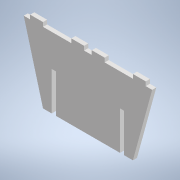
# Autodesk Inventor part: Base_Soporte
Saved by Autodesk Inventor 2022 (Build 260153000, 153)
## iProperties
Created: 2022-02-08
Part Number: Base_Soporte
Material: Generic
Document SubType Name: Modeling
Designer: katha
Density: 1 g/cm^3
Appearance: Default
Author: katha
Autodesk Inventor part; units mm, degrees
ref_plane "YZ Plane" through (0, 0, 0) normal (1, 0, 0) x (0, 1, 0)
ref_plane "XZ Plane" through (0, 0, 0) normal (0, 1, 0) x (-1, 0, 0)
ref_plane "XY Plane" through (0, 0, 0) normal (0, 0, 1) x (1, 0, 0)
sketch "Sketch1" plane through (0, 0, 0) normal (0, 0, 1) x (1, 0, 0)
  line L0 (49.5311, 184.3064) -> (52.7311, 184.3064) projected
  line L1 (105.9311, 184.3064) -> (102.7311, 184.3064) projected
  line L2 (105.9311, 181.1064) -> (102.7311, 181.1064) projected
  line L3 (49.5311, 181.1064) -> (52.7311, 181.1064) projected
  line L4 (77.7311, 181.1064) -> (77.7311, 126.1064) construction
  line L5 (77.7311, 126.1064) -> (112.7311, 126.1064)
  line L6 (77.7311, 181.1064) -> (127.7311, 181.1064)
  line L7 (112.7311, 126.1064) -> (127.7311, 181.1064)
  line L8 (105.9311, 126.1064) -> (105.9311, 156.1064)
  line L9 (105.9311, 156.1064) -> (102.7311, 156.1064)
  line L10 (102.7311, 156.1064) -> (102.7311, 126.1064)
  line L11 (105.9311, 181.1064) -> (105.9311, 45.0595) projected
  line L12 (77.7311, 126.1064) -> (42.7311, 126.1064)
  line L13 (77.7311, 181.1064) -> (27.7311, 181.1064)
  line L14 (42.7311, 126.1064) -> (27.7311, 181.1064)
  line L15 (49.5311, 126.1064) -> (49.5311, 156.1064)
  line L16 (49.5311, 156.1064) -> (52.7311, 156.1064)
  line L17 (52.7311, 156.1064) -> (52.7311, 126.1064)
  line L18 (80.7311, 181.1064) -> (80.7311, 184.3064)
  line L19 (80.7311, 184.3064) -> (90.7311, 184.3064)
  line L20 (90.7311, 184.3064) -> (90.7311, 181.1064)
  line L21 (74.7311, 181.1064) -> (74.7311, 184.3064)
  line L22 (74.7311, 184.3064) -> (64.7311, 184.3064)
  line L23 (64.7311, 184.3064) -> (64.7311, 181.1064)
  line L24 (51.1311, 156.1064) -> (51.1311, 169.2307) construction
  line L25 (32.7311, 181.1064) -> (32.7311, 184.3064)
  line L26 (32.7311, 184.3064) -> (42.7311, 184.3064)
  line L27 (42.7311, 184.3064) -> (42.7311, 181.1064)
  line L28 (122.7311, 181.1064) -> (122.7311, 184.3064)
  line L29 (122.7311, 184.3064) -> (112.7311, 184.3064)
  line L30 (112.7311, 184.3064) -> (112.7311, 181.1064)
  point P0 (0, 0)
  dimension "d0" = 55
  dimension "d1" = 35
  dimension "d2" = 50
  dimension "d3" = 25
  dimension "d4" = 30
  dimension "d5" = 3.2
  dimension "d6" = 3.2
  dimension "d7" = 10
  dimension "d8" = 3
  dimension "d11" = 3.2
  dimension "d12" = 10
  dimension "d13" = 5
  constraints: 52 end point, 14 symmetric about line, 8 point on line, 7 perpendicular, 4 vertical, 2 collinear, 2 horizontal, 1 midpoint
  measures "d0" distance of L4.start L4.end
  measures "d1" distance of L4.end L5.end
  measures "d2" distance of L4.start L6.end
  measures "d3" distance from line of L4 L2.end
  measures "d4" distance of L8.start L8.end
  measures "d5" distance between parallel lines of L10 L8
  measures "d6" distance of L18.start L18.end
  measures "d7" distance of L18.end L19.end
  measures "d8" distance from line of L4.start L18
  measures "d11" distance of L25.start L25.end
  measures "d12" distance of L25.end L26.end
  measures "d13" distance from line of L14.end L25
extrude "Extrusion1" add sketch "Sketch1" along normal mid plane 3.2 contours L11 L9 L10 L5 L12 L17 L16 L15 L14 L13 L3 L6 L2 | L6 L7 L5 L8 L11 | L30 L29 L28 L6 | L6 L18 L19 L20 | L13 L23 L22 L21 | L13 L25 L26 L27
body "Solid1"
